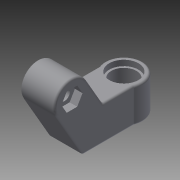
# Autodesk Inventor part: hub top
Saved by Autodesk Inventor 2013 (Build 170138000, 138)
## iProperties
Created: 2013-07-14
Part Number: hub top
Material: Generic
Document SubType Name: Modeling
Designer: employee
Density: 1 g/cm^3
Author: employee
Autodesk Inventor part; units mm, degrees
ref_plane "YZ Plane" through (0, 0, 0) normal (1, 0, 0) x (0, 1, 0)
ref_plane "XZ Plane" through (0, 0, 0) normal (0, 1, 0) x (-1, 0, 0)
ref_plane "XY Plane" through (0, 0, 0) normal (0, 0, 1) x (1, 0, 0)
sketch "Sketch1" plane through (0, 0, 0) normal (1, 0, 0) x (0, 1, 0)
  circle A0 centre (-50, 14) radius 4.05
  arc A1 (-39.1747, 20.25) -> (-60.8253, 7.75) centre (-50, 14) ccw
  line L0 (0, 0) -> (0, -25)
  line L1 (0, -25) -> (-41.9171, -25)
  line L2 (-41.9171, -25) -> (-60.8253, 7.75)
  line L3 (0, 0) -> (-27.4833, 0)
  line L4 (-27.4833, 0) -> (-39.1747, 20.25)
  dimension "d0" = 8.1
  dimension "d2" = 50
  dimension "d3" = 14
  dimension "d4" = 25
  dimension "d6" = 25
  dimension "d40" = 120
  constraints: 10 end point, 2 centre point, 2 parallel, 2 point on circle, 2 tangent, 1 coincident, 1 perpendicular, 1 vertical
  measures "d0" diameter of A0
  measures "d2" horizontal distance of L0.start A0.centre
  measures "d3" vertical distance of A0.centre L0.start
  measures "d4" diameter of A1
  measures "d6" distance of L0.start L0.end
  measures "d40" angle of L2 L1
extrude "Extrusion1" add sketch "Sketch1" along normal mid plane 25
sketch "Sketch2" plane through (-12.5, -27.4833, 0) normal (0, 0, 1) x (1, 0, 0)
  circle A0 centre (12.5, 27.4833) radius 12.5
  constraints: 1 centre point, 1 coincident
extrude "Extrusion2" add sketch "Sketch2" against normal up to surface (25 mm away)
sketch "Sketch13" plane through (-12.5, -27.4833, 0) normal (0, 0, 1) x (1, 0, 0)
  arc A0 (25, 27.4833) -> (0, 27.4833) centre (12.5, 27.4833) ccw projected
  circle A1 centre (12.5, 27.4833) radius 9.05
  dimension "d59" = 18.1
  constraints: 1 centre point, 1 coincident
  measures "d59" diameter of A1
extrude "Extrusion13" cut sketch "Sketch13" against normal through all
sketch "Sketch14" plane through (-12.5, -27.4833, 0) normal (0, 0, 1) x (1, 0, 0)
  circle A0 centre (12.5, 27.4833) radius 9.05 projected
  arc A1 (25, 27.4833) -> (0, 27.4833) centre (12.5, 27.4833) ccw projected
  circle A2 centre (12.5, 27.4833) radius 10.55
  dimension "d63" = 21.1
  constraints: 1 centre point, 1 coincident
  measures "d63" diameter of A2
extrude "Extrusion14" cut sketch "Sketch14" against normal blind 4
sketch "Sketch15" plane through (12.5, -41.9171, -25) normal (0, 0, -1) x (-1, 0, 0)
  circle A0 centre (12.5, 41.9171) radius 9.05 projected
  arc A1 (25, 41.9171) -> (0, 41.9171) centre (12.5, 41.9171) ccw projected
  circle A2 centre (12.5, 41.9171) radius 10.55
  dimension "d67" = 21.1
  constraints: 1 centre point, 1 coincident
  measures "d67" diameter of A2
extrude "Extrusion15" cut sketch "Sketch15" against normal blind 4
chamfer "Chamfer4" distance 1.5 angle 45 1 edges at (-9.05, 0, -21)
sketch "Sketch16" plane through (-12.5, -27.4833, 0) normal (0, 0, 1) x (1, 0, 0)
  circle A0 centre (12.5, 27.4833) radius 10.55 projected
  arc A1 (25, 27.4833) -> (0, 27.4833) centre (12.5, 27.4833) ccw projected
  circle A2 centre (12.5, 27.4833) radius 13.55
  dimension "d76" = 3
  constraints: 1 centre point, 1 coincident
  measures "d76" radial gap between concentric circles of A2 A0
extrude "Extrusion16" add sketch "Sketch16" against normal up to surface (25 mm away)
sketch "Sketch17" plane through (12.5, 0, 0) normal (1, 0, 0) x (0, 0, -1)
  arc A0 (-19.5, -40.4737) -> (-8.5, -59.5263) centre (-14, -50) ccw projected
  line L0 (-14, -42.379) -> (-7.4, -46.1895)
  line L1 (-7.4, -46.1895) -> (-7.4, -53.8105)
  line L2 (-7.4, -53.8105) -> (-14, -57.621)
  line L3 (-14, -57.621) -> (-20.6, -53.8105)
  line L4 (-20.6, -53.8105) -> (-20.6, -46.1895)
  line L5 (-20.6, -46.1895) -> (-14, -42.379)
  point P0 (0, 0)
  dimension "d80" = 13.2
  constraints: 12 end point, 1 coincident, 1 vertical alignment, 13 other
  measures "d80" distance between parallel lines of L1 L4
extrude "Extrusion17" cut sketch "Sketch17" against normal blind 5.5
sketch "Sketch18" plane through (12.5, -41.9171, -25) normal (0, 0, -1) x (-1, 0, 0)
  line L0 (25, -20.5829) -> (0, -20.5829) projected
  circle A0 centre (12.5, -20.5829) radius 8.5
  dimension "d83" = 17
  constraints: 1 centre point, 1 midpoint
  measures "d83" diameter of A0
extrude "Extrusion18" cut sketch "Sketch18" against normal through all
body "Solid1"
